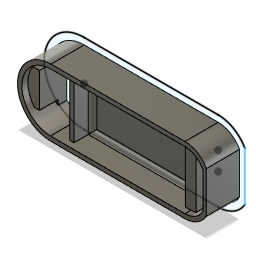
dictofun_case_bottom (Autodesk Fusion 360 design; units mm, degrees)
Autodesk Fusion 360 part; units mm, degrees
sketch "Sketch1" plane through (0, 0, 0) normal (0, 0, 1) x (1, 0, 0)
  line L0 (0, 0) -> (42, 0)
  line L1 (42, 0) -> (42, 13.5)
  line L2 (42, 13.5) -> (0, 13.5)
  line L3 (0, 13.5) -> (0, 0)
  arc A0 (6.7507, 13.5) -> (6.6112, 0) centre (6.7507, 6.7493) ccw
  arc A1 (42, 10.8) -> (37.8, 13.5) centre (37.8, 8.8833) ccw
  arc A2 (37.8, 0) -> (42, 2.7) centre (37.8, 4.6167) ccw
  arc A3 (6.7507, 14.4993) -> (6.7507, -1.0007) centre (6.7507, 6.7493) ccw
  line L4 (6.7507, 14.4993) -> (37.8, 14.4993)
  line L5 (6.7507, -1.0007) -> (37.8, -1.0007)
  arc A4 (42.7553, 11.526) -> (37.8, 14.4993) centre (37.8, 8.8833) ccw
  arc A5 (37.8, -1.0007) -> (42.7553, 1.971) centre (37.8, 4.6167) ccw
  line L6 (42.7553, 11.526) -> (42.7553, 1.971)
  dimension "d1" = 42
  dimension "d2" = 13.5
  dimension "d3" = 2.7
  dimension "d4" = 4.2
  dimension "d5" = 4.2
  dimension "d6" = 2.7
  dimension "d8" = 7.75
  constraint horizontal L0
  constraint vertical L1
  constraint horizontal L2
  constraint vertical L3
  constraint coincident L0.start L3.end
  constraint coincident L2 A0.start
  constraint tangent L3 A0
  constraint tangent L2 A0
  constraint tangent L2 A1
  constraint coincident L1 A1.start
  constraint coincident L2 A1.end
  constraint tangent L0 A2
  constraint coincident L1 A2.end
  constraint coincident L0 A2.start
  constraint coincident A0.centre A3.centre
  constraint tangent A3 L4
  constraint parallel L2 L4
  constraint tangent A3 L5
  constraint parallel L0 L5
  constraint coincident A1.centre A4.centre
  constraint coincident A2.centre A5.centre
  constraint parallel L1 L6
  constraint coincident L0 A0.end
  constraint tangent L4 A4
  constraint tangent L5 A5
  measures "d1" distance of L0.start L0.end
  measures "d2" distance of L0.start L2.end
  measures "d3" distance of L1.end A1.start
  measures "d4" distance of L1.end A1.end
  measures "d5" distance of L0.end A2.start
  measures "d6" distance of L0.end A2.end
  measures "d8" radius of A3
extrude "Extrude1" add sketch "Sketch1" along normal blind 5.7 contours L0 A3 L5 A5 | L0 L3 A0 A3 | L0 L1 A2 A5 | L3 A3 | L2 L3 A0 A3 | L1 A4 A5 L6 | L2 A3 L4 A4 | L1 L2 A1 A4
sketch "Sketch2" plane through (0, 0, 0) normal (0, 0, -1) x (-1, 0, 0)
  arc A0 (-42, 2.7) -> (-37.8, 0) centre (-37.8, 4.6167) ccw
  line L0 (-42, 2.7) -> (-42, 10.8)
  arc A1 (-37.8, 13.5) -> (-42, 10.8) centre (-37.8, 8.8833) ccw
  line L1 (-37.8, 13.5) -> (-6.7507, 13.5)
  arc A2 (-6.6112, 0) -> (-6.7507, 13.5) centre (-6.7507, 6.7493) ccw
  line L2 (-6.6112, 0) -> (-37.8, 0)
  arc A3 (-6.7507, -1.0007) -> (-6.7507, 14.4993) centre (-6.7507, 6.7493) ccw
  line L3 (-6.7507, 14.4993) -> (-37.8, 14.4993)
  arc A4 (-37.8, 14.4993) -> (-42.7553, 11.526) centre (-37.8, 8.8833) ccw
  line L4 (-42.7553, 11.526) -> (-42.7553, 1.971)
  arc A5 (-42.7553, 1.971) -> (-37.8, -1.0007) centre (-37.8, 4.6167) ccw
  line L5 (-37.8, -1.0007) -> (-6.7507, -1.0007)
extrude "Extrude2" add sketch "Sketch2" along normal blind 2 contours A0 L0 A1 L1 A2 L2 | A3 L3 A4 L4 A5 L5
sketch "Sketch3" plane through (0, 0, 0) normal (0, 0, 1) x (1, 0, 0)
  line L0 (42, 2.7) -> (42, 10.8)
  arc A0 (42, 10.8) -> (37.8, 13.5) centre (37.8, 8.8833) ccw
  line L1 (37.8, 13.5) -> (6.7507, 13.5)
  arc A1 (6.7507, 13.5) -> (6.6112, 0) centre (6.7507, 6.7493) ccw
  line L2 (6.6112, 0) -> (37.8, 0)
  arc A2 (37.8, 0) -> (42, 2.7) centre (37.8, 4.6167) ccw
  line L3 (36.5, 13.5) -> (39, 13.5)
  line L4 (39, 13.5) -> (39, 0.1148)
  line L5 (37.8, 0) -> (36.5, 0)
  line L6 (36.5, 0) -> (36.5, 13.5)
  line L7 (0, 10.5) -> (2.7, 10.5)
  line L8 (2.7, 10.5) -> (2.7, 2.5)
  line L9 (2.7, 2.5) -> (0, 2.5)
  line L10 (0, 2.5) -> (0, 10.5)
  dimension "d13" = 2.5
  dimension "d14" = 2.7
  dimension "d15" = 3
  constraint horizontal L3
  constraint vertical L4
  constraint horizontal L5
  constraint vertical L6
  constraint coincident A2 L2.end
  constraint coincident L1 L3.start
  constraint collinear L2 L5
  constraint horizontal L7
  constraint vertical L8
  constraint horizontal L9
  constraint vertical L10
  constraint tangent A1 L10
  measures "d13" distance of L3.start L3.end
  measures "d14" distance of L8 L10
  measures "d15" distance of L0 L4
extrude "Extrude3" add sketch "Sketch3" along normal blind 4.3 contours A0 L1 L2 A2 L3 L4 L5 L6 | A1 L7 L8 L9
sketch "Sketch4" plane through (0, 0, 0) normal (0, 0, 1) x (1, 0, 0)
  line L0 (36.5, 0) -> (36.5, 13.5)
  line L1 (36.5, 13.5) -> (6.7507, 13.5)
  arc A0 (6.7507, 13.5) -> (1.1378, 10.5) centre (6.7507, 6.7493) ccw
  line L2 (1.1378, 10.5) -> (2.7, 10.5)
  line L3 (2.7, 10.5) -> (2.7, 2.5)
  line L4 (2.7, 2.5) -> (1.5052, 2.5)
  arc A1 (1.5052, 2.5) -> (6.6112, 0) centre (6.7507, 6.7493) ccw
  line L5 (6.6112, 0) -> (36.5, 0)
  line L6 (2.7, 10.5) -> (2.7, 12.1496)
  line L7 (2.7, 2.5) -> (2.7, 1.3489)
  line L8 (9.7, 13.5) -> (9.7, 0)
  dimension "d20" = 7
  constraint coincident L2.end L3.start
  constraint coincident A0 L6.end
  constraint perpendicular L2 L6
  constraint coincident L3.end L4.start
  constraint coincident A1 L7.end
  constraint perpendicular L4 L7
  constraint coincident L1 L8.start
  constraint perpendicular L1 L8
  measures "d20" distance of L3 L8
extrude "Extrude4" cut sketch "Sketch4" against normal blind 2 contours L1 A0 L3 A1 L5 L6 L7 L8
sketch "Sketch5" plane through (0, 0, 0) normal (0, 0, 1) x (1, 0, 0)
  line L0 (9.7, 13.5) -> (9.7, 0)
  line L1 (9.7, 0) -> (36.5, 0)
  line L2 (36.5, 0) -> (36.5, 13.5)
  line L3 (36.5, 13.5) -> (9.7, 13.5)
  line L4 (9.7, 0) -> (10.7, 0)
  line L5 (10.7, 0) -> (10.7, 13.5)
  line L6 (10.7, 13.5) -> (9.7, 13.5)
  line L7 (9.7, 13.5) -> (9.7, 0)
  dimension "d23" = 1
  constraint horizontal L4
  constraint vertical L5
  constraint horizontal L6
  constraint vertical L7
  constraint coincident L0.end L1.start
  measures "d23" distance of L5 L7
extrude "Extrude5" add sketch "Sketch5" along normal blind 4.3 contours L0 L1 L3 L4 L5 L6 L7
fillet "Fillet1" radius 1 4 edges at (23.6, 13.5, 0) (23.6, 0, 0) (42, 6.75, 0) (10.7, 6.75, 0)
fillet "Fillet2" [suppressed]
sketch "Sketch6" plane through (0, 0, -2) normal (0, 0, -1) x (-1, 0, 0)
  line L0 (-2.7, 12.1496) -> (-2.7, 1.3489)
  arc A0 (-6.6112, 0) -> (-2.7, 1.3489) centre (-6.7507, 6.7493) ccw
  line L1 (-6.6112, 0) -> (-9.7, 0)
  line L2 (-9.7, 0) -> (-9.7, 13.5)
  line L3 (-9.7, 13.5) -> (-6.7507, 13.5)
  arc A1 (-2.7, 12.1496) -> (-6.7507, 13.5) centre (-6.7507, 6.7493) ccw
  line L4 (-37.8, -1.0007) -> (-6.7507, -1.0007)
  arc A2 (-6.7507, -1.0007) -> (-6.7507, 14.4993) centre (-6.7507, 6.7493) ccw
  line L5 (-6.7507, 14.4993) -> (-37.8, 14.4993)
  arc A3 (-37.8, 14.4993) -> (-42.7553, 11.526) centre (-37.8, 8.8833) ccw
  line L6 (-42.7553, 11.526) -> (-42.7553, 1.971)
  arc A4 (-42.7553, 1.971) -> (-37.8, -1.0007) centre (-37.8, 4.6167) ccw
  arc A5 (-6.7511, -2.5007) -> (-6.7507, 15.9993) centre (-6.7507, 6.7493) ccw
  arc A6 (-37.8, 15.9993) -> (-43.9996, 12.3764) centre (-37.8, 8.8833) ccw
  arc A7 (-43.9996, 1.1236) -> (-37.8003, -2.4993) centre (-37.8, 4.6167) ccw
  line L7 (-43.9996, 12.3764) -> (-43.9996, 1.1236)
  line L8 (-37.8, 15.9993) -> (-6.7507, 15.9993)
  line L9 (-6.7511, -2.5007) -> (-37.8003, -2.4993)
  dimension "d30" = 9.25
  dimension "d31" = 5.6159
  dimension "d32" = 7.116
  dimension "d33" = 7.116
  constraint coincident A0.centre A1.centre
  constraint coincident A3.centre A6.centre
  constraint coincident A4.centre A7.centre
  constraint parallel L6 L7
  constraint tangent A6 L8
  constraint tangent A5 L8
  constraint tangent A5 L9
  constraint tangent A7 L9
  measures "d30" radius of A5
  measures "d31" radius of A3
  measures "d32" radius of A6
  measures "d33" radius of A7
extrude "Extrude6" [suppressed]
fillet "Fillet3" [suppressed]
sketch "Sketch7" plane through (0, 0, 0) normal (0, 0, 1) x (1, 0, 0)
  line L0 (11.7, 1) -> (36.5, 1)
  line L1 (36.5, 1) -> (36.5, 12.5)
  line L2 (36.5, 12.5) -> (11.7, 12.5)
  line L3 (11.7, 12.5) -> (11.7, 1)
  circle A0 centre (36.5, 9.25) radius 1.65
  circle A1 centre (36.5, 4.25) radius 1.65
  line L4 (42, 10.8) -> (42, 2.7)
  line L5 (42.7553, 1.971) -> (42.7553, 11.526)
  line L6 (6.7507, 13.5) -> (37.8, 13.5)
  dimension "d38" = 3.3
  dimension "d39" = 3.3
  dimension "d40" = 5.5
  dimension "d42" = 5.5
  dimension "d43" = 5
  dimension "d44" = 4.25
  measures "d38" diameter of A0
  measures "d39" diameter of A1
  measures "d40" distance of A0.centre L4
  measures "d42" distance of A1.centre L4
  measures "d43" distance of A0.centre A1.centre
  measures "d44" distance of A0.centre L6
extrude "Extrude7" [suppressed]
sketch "Sketch8" plane through (0, 0, 0) normal (0, 0, 1) x (1, 0, 0)
  line L0 (41, 1.289) -> (41, 12.211)
  arc A0 (41, 12.211) -> (39, 13.3413) centre (37.8, 8.8833) ccw
  line L1 (39, 13.3413) -> (39, 0.1587)
  arc A1 (39, 0.1587) -> (41, 1.289) centre (37.8, 4.6167) ccw
  circle A2 centre (40, 8.25) radius 1
  circle A3 centre (40, 5.25) radius 1
  line L2 (42, 10.8) -> (42, 2.7)
  line L3 (6.7507, 13.5) -> (37.8, 13.5)
  dimension "d49" = 2
  dimension "d50" = 2
  dimension "d51" = 2
  dimension "d52" = 5.25
  dimension "d53" = 3
  constraint vertical A2.centre A3.centre
  measures "d49" diameter of A2
  measures "d50" diameter of A3
  measures "d51" distance of A2.centre L2
  measures "d52" distance of A2.centre L3
  measures "d53" distance of A2.centre A3.centre
extrude "Extrude8" [suppressed]
sketch "Sketch9" plane through (0, 0, -2) normal (0, 0, -1) x (-1, 0, 0)
  circle A0 centre (-40, 8.25) radius 1
  circle A1 centre (-40, 5.25) radius 1
  arc A2 (-37.8, 15.9993) -> (-43.9996, 12.3764) centre (-37.8, 8.8833) ccw
  line L0 (-43.9996, 12.3764) -> (-43.9996, 1.1236)
  arc A3 (-43.9996, 1.1236) -> (-37.8003, -2.4993) centre (-37.8, 4.6167) ccw
  line L1 (-37.8003, -2.4993) -> (-6.7511, -2.5007)
  arc A4 (-6.7511, -2.5007) -> (-6.7507, 15.9993) centre (-6.7507, 6.7493) ccw
  line L2 (-6.7507, 15.9993) -> (-37.8, 15.9993)
  line L3 (-2.7, 12.1496) -> (-2.7, 1.3489)
  arc A5 (-6.6112, 0) -> (-2.7, 1.3489) centre (-6.7507, 6.7493) ccw
  line L4 (-6.6112, 0) -> (-9.7, 0)
  line L5 (-9.7, 0) -> (-9.7, 13.5)
  line L6 (-9.7, 13.5) -> (-6.7507, 13.5)
  arc A6 (-2.7, 12.1496) -> (-6.7507, 13.5) centre (-6.7507, 6.7493) ccw
  arc A7 (-45.8001, 15.9993) -> (-50.741, 11.0584) centre (-45.8001, 11.0584) ccw
  arc A8 (-50.741, 2.442) -> (-45.8003, -2.499) centre (-45.8001, 2.442) ccw
  line L7 (-37.8003, -2.4993) -> (-45.8003, -2.499)
  line L8 (-37.8, 15.9993) -> (-45.8001, 15.9993)
  line L9 (-50.741, 11.0584) -> (-50.741, 2.442)
  line L10 (-43.9996, 1.1236) -> (-45.4996, 1.1236)
  arc A9 (-47.9996, 3.6236) -> (-45.4996, 1.1236) centre (-45.4996, 3.6236) ccw
  line L11 (-47.9996, 9.8764) -> (-47.9996, 3.6236)
  line L12 (-43.9996, 12.3764) -> (-45.4996, 12.3764)
  arc A10 (-45.4996, 12.3764) -> (-47.9996, 9.8764) centre (-45.4996, 9.8764) ccw
  dimension "d56" = 8
  dimension "d57" = 4
  dimension "d58" = 1.5
  dimension "d59" = 2.5
  dimension "d60" = 2.5
  constraint coincident A3.end L1.start
  constraint coincident A2.start L2.end
  constraint collinear L2 L8
  constraint collinear L1 L7
  constraint vertical A7.end A8.start
  constraint vertical A7.centre A8.centre
  constraint tangent A7 L8
  constraint tangent A8 L7
  constraint tangent A7 L9
  constraint tangent A8 L9
  constraint coincident L0.end A3.start
  constraint perpendicular L0 L10
  constraint tangent A7 A9
  constraint parallel L9 L11
  constraint tangent L10 A9
  constraint tangent A9 L11
  constraint coincident A2.end L0.start
  constraint perpendicular L0 L12
  constraint tangent L11 A10
  constraint tangent L12 A10
  measures "d56" horizontal distance of A8.end A3.end
  measures "d57" distance of L0 L11
  measures "d58" distance of L0.end L10.end
  measures "d59" radius of A10
  measures "d60" radius of A9
extrude "Extrude9" [suppressed]
fillet "Fillet4" [suppressed]
sketch "Sketch10" plane through (0, 0, -2) normal (0, 0, -1) x (-1, 0, 0)
  line L0 (-2.7, 12.1496) -> (-2.7, 1.3489)
  arc A0 (-6.6112, 0) -> (-2.7, 1.3489) centre (-6.7507, 6.7493) ccw
  line L1 (-6.6112, 0) -> (-9.7, 0)
  line L2 (-9.7, 0) -> (-9.7, 13.5)
  line L3 (-9.7, 13.5) -> (-6.7507, 13.5)
  arc A1 (-2.7, 12.1496) -> (-6.7507, 13.5) centre (-6.7507, 6.7493) ccw
  line L4 (-43.9996, 1.1236) -> (-45.4996, 1.1236)
  arc A2 (-47.9996, 3.6236) -> (-45.4996, 1.1236) centre (-45.4996, 3.6236) ccw
  line L5 (-47.9996, 3.6236) -> (-47.9996, 9.8764)
  arc A3 (-45.4996, 12.3764) -> (-47.9996, 9.8764) centre (-45.4996, 9.8764) ccw
  line L6 (-45.4996, 12.3764) -> (-43.9996, 12.3764)
  line L7 (-43.9996, 12.3764) -> (-43.9996, 1.1236)
  circle A4 centre (-40, 5.25) radius 1
  circle A5 centre (-40, 8.25) radius 1
  arc A6 (-6.751, -0.5007) -> (-6.7507, 13.9993) centre (-6.7507, 6.7493) ccw
  line L8 (-6.7507, 13.9993) -> (-37.8, 13.9993)
  line L9 (-37.8, 13.9993) -> (-45.8001, 13.9993)
  arc A7 (-45.8001, 13.9993) -> (-48.741, 11.0584) centre (-45.8001, 11.0584) ccw
  line L10 (-48.741, 11.0584) -> (-48.741, 2.442)
  arc A8 (-48.741, 2.442) -> (-45.8002, -0.499) centre (-45.8001, 2.442) ccw
  line L11 (-45.8002, -0.499) -> (-37.8002, -0.4993)
  line L12 (-37.8002, -0.4993) -> (-6.751, -0.5007)
  line L13 (-43.9996, 9.45) -> (-41, 9.45)
  line L14 (-41, 9.45) -> (-41, 9.05)
  line L15 (-41, 9.05) -> (-43.9996, 9.05)
  line L16 (-43.9996, 9.05) -> (-43.9996, 9.45)
  line L17 (-43.9996, 7.45) -> (-41, 7.45)
  line L18 (-41, 7.45) -> (-41, 7.05)
  line L19 (-41, 7.05) -> (-43.9996, 7.05)
  line L20 (-43.9996, 7.05) -> (-43.9996, 7.45)
  line L21 (-43.9996, 6.45) -> (-41, 6.45)
  line L22 (-41, 6.45) -> (-41, 6.05)
  line L23 (-41, 6.05) -> (-43.9996, 6.05)
  line L24 (-43.9996, 6.05) -> (-43.9996, 6.45)
  line L25 (-43.9996, 4.45) -> (-41, 4.45)
  line L26 (-41, 4.45) -> (-41, 4.05)
  line L27 (-41, 4.05) -> (-43.9996, 4.05)
  line L28 (-43.9996, 4.05) -> (-43.9996, 4.45)
  dimension "d65" = 1.6
  dimension "d67" = 1.6
  dimension "d68" = 0.8
  dimension "d69" = 0.8
  dimension "d70" = 0.4
  dimension "d71" = 0.4
  dimension "d72" = 0.4
  dimension "d73" = 0.4
  constraint horizontal L13
  constraint vertical L14
  constraint horizontal L15
  constraint vertical L16
  constraint coincident L7 L13.start
  constraint horizontal L17
  constraint vertical L18
  constraint horizontal L19
  constraint vertical L20
  constraint coincident L7 L17.start
  constraint horizontal L21
  constraint vertical L22
  constraint horizontal L23
  constraint vertical L24
  constraint coincident L7 L21.start
  constraint horizontal L25
  constraint vertical L26
  constraint horizontal L27
  constraint vertical L28
  constraint coincident L7 L25.start
  measures "d65" distance of L23 L25
  measures "d67" distance of L15 L17
  measures "d68" distance of A5.centre L15
  measures "d69" distance of A4.centre L23
  measures "d70" distance of L13 L15
  measures "d71" distance of L17 L19
  measures "d72" distance of L21 L23
  measures "d73" distance of L25 L27
extrude "Extrude10" [suppressed]
